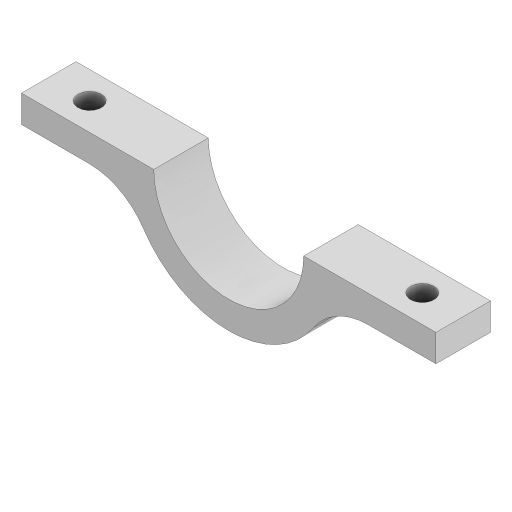
# Autodesk Inventor part: Part1
Saved by Autodesk Inventor 2023.3 (Build 273359000, 359)
## iProperties
Created: 2025-06-02
Part Number: Part1
Material: Generic
Document SubType Name: Modeling
Designer: David Zindović
Density: 1 g/cm^3
Appearance: Default
Author: David Zindović
Autodesk Inventor part; units mm, degrees
ref_plane "YZ Plane" through (0, 0, 0) normal (1, 0, 0) x (0, 1, 0)
ref_plane "XZ Plane" through (0, 0, 0) normal (0, 1, 0) x (-1, 0, 0)
ref_plane "XY Plane" through (0, 0, 0) normal (0, 0, 1) x (1, 0, 0)
sketch "Sketch1" plane through (0, 0, 0) normal (0, 0, 1) x (1, 0, 0)
  circle A0 centre (0, 0) radius 13.75
  circle A1 centre (0, 0) radius 18.75
  line L0 (-18.75, 0) -> (-38, 0)
  line L1 (-38, 0) -> (-38, -5)
  line L2 (-38, -5) -> (-18.75, -5)
  line L3 (-18.75, -5) -> (-18.75, 0)
  line L4 (-18.75, -5) -> (-13.75, -5)
  line L5 (-13.75, -5) -> (-13.75, 0)
  line L6 (-13.75, 0) -> (-18.75, 0)
  line L7 (-18.75, 0) -> (-18.75, -5)
  line L8 (18.75, 0) -> (38, 0)
  line L9 (38, 0) -> (38, -5)
  line L10 (38, -5) -> (18.75, -5)
  line L11 (18.75, -5) -> (18.75, 0)
  line L12 (18.75, -5) -> (13.75, -5)
  line L13 (13.75, -5) -> (13.75, 0)
  line L14 (13.75, 0) -> (18.75, 0)
  line L15 (18.75, 0) -> (18.75, -5)
  point P0 (-18.071, -5)
  point P1 (18.071, -5)
  dimension "d0" = 27.5
  dimension "d1" = 5
  dimension "d2" = 5
  dimension "d3" = 19.25
  dimension "d4" = 19.25
  dimension "d5" = 5
  constraints: 32 end point, 8 parallel, 4 horizontal, 4 perpendicular, 4 point on circle, 2 centre point, 1 coincident, 1 point on line
  measures "d0" diameter of A0
  measures "d1" radial gap between concentric circles of A0 A1
  measures "d2" distance of L1.end L0.end
  measures "d3" distance of L1.end L2.end
  measures "d4" distance of L9.end L10.end
  measures "d5" distance of L8.end L9.end
extrude "Extrusion1" add sketch "Sketch1" along normal blind 10 contours L13 L12 A1 L4 L5 A0 | L14 A1 L12 L13 | L5 L4 A1 L6 | L11 L12 A1 | L8 L9 L10 L11 | L3 L2 L1 L0 | A1 L4 L3
sketch "Sketch2" plane through (-38, -5, 0) normal (0, -1, 0) x (1, 0, 0)
  line L0 (0, 0) -> (19.929, 0) projected
  line L1 (19.929, 0) -> (19.929, 10) projected
  line L2 (0, 10) -> (19.929, 10) projected
  line L3 (0, 0) -> (0, 10) projected
  line L4 (56.071, 0) -> (76, 0) projected
  line L5 (76, 0) -> (76, 10) projected
  line L6 (56.071, 10) -> (76, 10) projected
  line L7 (56.071, 0) -> (56.071, 10) projected
  circle A0 centre (7.5, 5) radius 2.15
  circle A1 centre (68.5, 5) radius 2.15
  line L8 (0, 0) -> (0, 10) projected
  line L9 (76, 0) -> (76, 10) projected
  point P0 (38, 0)
  point P1 (9.9645, 10)
  point P2 (0, 5)
  point P3 (66.0355, 10)
  point P4 (76, 5)
  point P5 (0, 5)
  point P6 (0, 5)
  point P7 (76, 5)
  point P8 (76, 5)
  dimension "d8" = 4.3
  dimension "d9" = 4.3
  dimension "d13" = 7.5
  dimension "d14" = 7.5
  constraints: 8 midpoint, 2 centre point, 2 horizontal alignment
  measures "d8" diameter of A0
  measures "d9" diameter of A1
  measures "d13" distance of point (0, 5) A0.centre
  measures "d14" distance of point (76, 5) A1.centre
extrude "Extrusion2" cut sketch "Sketch2" against normal up to surface (5 mm away) contours A0 | A1
fillet "Fillet1" radius 12 2 edges at (-18.071, -5, 5) (18.071, -5, 5)
equation "\"d4\" = d3"
body "Solid1"
